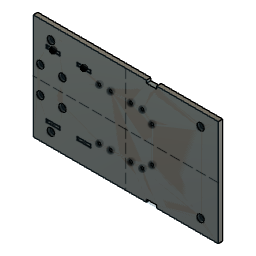
minibot v2 (Autodesk Fusion 360 design; units mm, degrees)
Autodesk Fusion 360 part; units mm, degrees
sketch "Sketch1" plane through (0, 0, 0) normal (0, 0, 1) x (1, 0, 0)
  line L0 (-105, 60) -> (105, 60)
  line L1 (105, 60) -> (105, -60)
  line L2 (105, -60) -> (-105, -60)
  line L3 (-105, -60) -> (-105, 60)
  line L4 (-105, 60) -> (105, -60) construction
  line L5 (105, 60) -> (-105, -60) construction
  dimension "d1" = 210
  dimension "d2" = 120
  constraint horizontal L0
  constraint perpendicular L0 L1
  constraint parallel L0 L2
  constraint parallel L1 L3
  constraint coincident L4 origin
  constraint coincident L5 origin
  measures "d1" distance of L1.end L2.end
  measures "d2" distance of L0.end L1.end
extrude "Extrude1" add sketch "Sketch1" along normal blind 5
sketch "Sketch2" plane through (0, 0, 5) normal (0, 0, 1) x (1, 0, 0)
  line L0 (-105, -60) -> (105, -60)
  line L1 (105, -60) -> (105, 60)
  line L2 (105, 60) -> (-105, 60)
  line L3 (-105, 60) -> (-105, -60)
  line L4 (0, 60) -> (0, -60) construction
  line L5 (105, 0) -> (-105, 0) construction
  line L6 (-75, 35) -> (-90, 35)
  line L7 (-90, 35) -> (-90, 38)
  line L8 (-90, 38) -> (-75, 38)
  line L9 (-75, 38) -> (-75, 35)
  line L10 (-75, 35) -> (-90, 38) construction
  line L11 (-90, 35) -> (-75, 38) construction
  line L12 (-55, 38) -> (-40, 38)
  line L13 (-40, 38) -> (-40, 35)
  line L14 (-40, 35) -> (-55, 35)
  line L15 (-55, 35) -> (-55, 38)
  line L16 (-55, 38) -> (-40, 35) construction
  line L17 (-40, 38) -> (-55, 35) construction
  line L18 (-40, -38) -> (-40, -35)
  line L19 (-55, -38) -> (-40, -35) construction
  line L20 (-40, -35) -> (-55, -35)
  line L21 (-55, -35) -> (-55, -38)
  line L22 (-55, -38) -> (-40, -38)
  line L23 (-40, -38) -> (-55, -35) construction
  line L24 (-75, -38) -> (-75, -35)
  line L25 (-90, -38) -> (-75, -38)
  line L26 (-90, -35) -> (-75, -38) construction
  line L27 (-75, -35) -> (-90, -38) construction
  line L28 (-75, -35) -> (-90, -35)
  line L29 (-90, -35) -> (-90, -38)
  point P0 (-85, 45)
  point P1 (85, 45)
  point P2 (30, 20)
  point P3 (19, 29)
  point P4 (6, 29)
  point P5 (-17, 29)
  point P6 (-30, 29)
  point P7 (-82.5, 36.5)
  point P8 (-47.5, 36.5)
  point P9 (-82.5, 36.5)
  point P10 (-47.5, 36.5)
  point P11 (-97, 15)
  point P12 (-72, 15)
  point P13 (85, -45)
  point P14 (30, -20)
  point P15 (19, -29)
  point P16 (6, -29)
  point P17 (-17, -29)
  point P18 (-30, -29)
  point P19 (-85, -45)
  point P20 (-97, -15)
  point P21 (-72, -15)
  dimension "d5" = 15
  dimension "d6" = 20
  dimension "d7" = 15
  dimension "d8" = 20
  dimension "d9" = 75
  dimension "d10" = 40
  dimension "d11" = 31
  dimension "d12" = 31
  dimension "d13" = 31
  dimension "d14" = 31
  dimension "d15" = 86
  dimension "d16" = 49
  dimension "d17" = 13
  dimension "d18" = 13
  dimension "d19" = 22.5
  dimension "d20" = 23.5
  dimension "d21" = 35
  dimension "d22" = 23.5
  dimension "d23" = 15
  dimension "d24" = 3
  dimension "d25" = 15
  dimension "d26" = 3
  dimension "d27" = 8
  dimension "d28" = 45
  dimension "d29" = 45
  dimension "d30" = 25
  constraint midpoint L2 L4.start
  constraint midpoint L0 L4.end
  constraint midpoint L1 L5.start
  constraint midpoint L3 L5.end
  constraint horizontal L6
  constraint perpendicular L6 L7
  constraint parallel L6 L8
  constraint parallel L7 L9
  constraint coincident L10 P9
  constraint coincident L11 P9
  constraint coincident P9 P7
  constraint horizontal L12
  constraint perpendicular L12 L13
  constraint parallel L12 L14
  constraint parallel L13 L15
  constraint coincident L16 P10
  constraint coincident L17 P10
  constraint coincident P10 P8
  constraint symmetric P0 L5 P19
  constraint symmetric P1 L5 P13
  constraint symmetric L5 P2 P14
  constraint symmetric L5 P3 P15
  constraint symmetric L5 P4 P16
  constraint symmetric L5 P5 P17
  constraint symmetric L5 P6 P18
  constraint symmetric L5 L6.start L24.end
  constraint symmetric L5 L6.end L26.start
  constraint symmetric L5 L7.end L25.start
  constraint symmetric L5 L8.end L24.start
  constraint symmetric L5 L12.start L19.start
  constraint symmetric L5 L12.end L18.start
  constraint symmetric L5 L13.end L18.end
  constraint symmetric L5 L14.end L20.end
  constraint symmetric L5 P11 P20
  constraint symmetric L5 P12 P21
  measures "d5" distance of L2 P0
  measures "d6" distance of L3 P0
  measures "d7" distance of L2 P1
  measures "d8" distance of L1 P1
  measures "d9" distance of L1 P2
  measures "d10" distance of L2 P2
  measures "d11" distance of L2 P3
  measures "d12" distance of L2 P4
  measures "d13" distance of L2 P5
  measures "d14" distance of L2 P6
  measures "d15" distance of L1 P3
  measures "d16" distance of P3 P6
  measures "d17" distance of P5 P6
  measures "d18" distance of P3 P4
  measures "d19" distance of L3 P9
  measures "d20" distance of L2 P9
  measures "d21" horizontal distance of P9 P10
  measures "d22" distance of L2 P10
  measures "d23" distance of L7.end L8.end
  measures "d24" distance of L6.end L7.end
  measures "d25" distance of L13.end L14.end
  measures "d26" distance of L12.end L13.end
  measures "d27" distance of L3 P11
  measures "d28" distance of L2 P11
  measures "d29" distance of L2 P12
  measures "d30" distance of P11 P12
extrude "Extrude2" cut sketch "Sketch2" against normal up to surface (5 mm away) contours L6 L7 L8 L9 | L12 L13 L14 L15 | L18 L20 L21 L22 | L24 L25 L28 L29
hole "Hole1" at (-85, 45, 5) at (85, 45, 5) at (-97, 15, 5) at (-72, 15, 5) at (-72, -15, 5) at (-97, -15, 5) at (-85, -45, 5) at (85, -45, 5) direction (0, 0, -1) diameter 3 depth 5 tip angle 180 counterbore diameter 8 counterbore depth 3
sketch "Sketch3" plane through (0, 0, 0) normal (0, 0, -1) x (-1, 0, 0)
  circle A0 centre (85, -45) radius 1.5
  circle A1 centre (72, -15) radius 1.5
  circle A2 centre (97, 15) radius 1.5
  circle A3 centre (85, 45) radius 1.5
  circle A4 centre (-85, 45) radius 1.5
  circle A5 centre (72, 15) radius 1.5
  circle A6 centre (97, -15) radius 1.5
  circle A7 centre (-85, -45) radius 1.5
  line L0 (75, 35) -> (75, 38)
  line L1 (75, 38) -> (90, 38)
  line L2 (90, 38) -> (90, 35)
  line L3 (90, 35) -> (75, 35)
  line L4 (75, -35) -> (90, -35)
  line L5 (90, -35) -> (90, -38)
  line L6 (90, -38) -> (75, -38)
  line L7 (75, -38) -> (75, -35)
  line L8 (55, 38) -> (55, 35)
  line L9 (55, 35) -> (40, 35)
  line L10 (40, 35) -> (40, 38)
  line L11 (40, 38) -> (55, 38)
  line L12 (55, -35) -> (55, -38)
  line L13 (55, -38) -> (40, -38)
  line L14 (40, -38) -> (40, -35)
  line L15 (40, -35) -> (55, -35)
  line L16 (-105, -60) -> (105, -60)
  line L17 (105, -60) -> (105, 60)
  line L18 (105, 60) -> (-105, 60)
  line L19 (-105, 60) -> (-105, -60)
  point P0 (-19, 29)
  point P1 (-30, 20)
  point P2 (-6, 29)
  point P3 (17, 29)
  point P4 (30, 29)
  point P5 (30, -29)
  point P6 (17, -29)
  point P7 (-6, -29)
  point P8 (-19, -29)
  point P9 (-30, -20)
hole "Hole3" at (-30, 29, 0) at (-17, 29, 0) at (6, 29, 0) at (19, 29, 0) at (30, 20, 0) at (30, -20, 0) at (19, -29, 0) at (6, -29, 0) at (-17, -29, 0) at (-30, -29, 0) direction (0, 0, 1) diameter 3 depth 5 tip angle 180 counterbore diameter 8 counterbore depth 3
sketch "Sketch5" plane through (0, 0, 5) normal (0, 0, 1) x (1, 0, 0)
  line L0 (-105, 60) -> (105, 60)
  line L1 (23.5, 60) -> (35, 60)
  line L2 (35, 60) -> (35, 57)
  line L3 (35, 57) -> (23.5, 57)
  line L4 (23.5, 57) -> (23.5, 60)
  line L5 (105, -60) -> (105, 60)
  line L6 (105, 0) -> (-105, 0)
  line L7 (23.5, -60) -> (35, -60)
  line L8 (23.5, -57) -> (23.5, -60)
  line L9 (35, -57) -> (23.5, -57)
  line L10 (35, -60) -> (35, -57)
  point P0 (35, 60)
  point P1 (105, 60)
  point P2 (23.5, 60)
  dimension "d49" = 70
  dimension "d50" = 11.5
  dimension "d51" = 3
  dimension "d52" = 70
  constraint coincident P0 L0
  constraint coincident L0 P2
  constraint horizontal L1
  constraint vertical L2
  constraint horizontal L3
  constraint vertical L4
  constraint coincident P2 L1.start
  constraint symmetric P2 L6 L7.start
  constraint symmetric P0 L6 L7.end
  constraint symmetric L2.end L6 L9.start
  constraint symmetric L3.end L6 L8.start
  measures "d49" distance of P0 L0.end
  measures "d50" distance of P0 P2
  measures "d51" distance of P2 L3.end
  measures "d52" distance of L2 L5
extrude "Extrude3" cut sketch "Sketch5" against normal up to surface (5 mm away)
